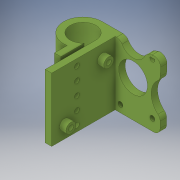
# Autodesk Inventor part: motor mount 2
Saved by Autodesk Inventor 2018 (Build 220112000, 112)
## iProperties
Created: 2017-11-21
Part Number: motor mount 2
Material: ABS Plastic
Document SubType Name: Modeling
Designer: prakhar
Density: 1.06 g/cm^3
Appearance: Olive Green
Author: prakhar
Autodesk Inventor part; units mm, degrees
ref_plane "YZ Plane" through (0, 0, 0) normal (1, 0, 0) x (0, 1, 0)
ref_plane "XZ Plane" through (0, 0, 0) normal (0, 1, 0) x (-1, 0, 0)
ref_plane "XY Plane" through (0, 0, 0) normal (0, 0, 1) x (1, 0, 0)
sketch "Sketch1" plane through (0, 0, 0) normal (1, 0, 0) x (0, 1, 0)
  line L0 (19.8793, 20.7795) -> (-17.4785, 20.7795)
  line L1 (-17.4785, 20.7795) -> (-17.4785, -16.5784)
  line L2 (-17.4785, -16.5784) -> (19.8793, -16.5784)
  line L3 (19.8793, -16.5784) -> (19.8793, 20.7795)
  circle A0 centre (19.8793, 20.7795) radius 4.8895
  circle A1 centre (19.8793, -16.5784) radius 4.8895
  circle A2 centre (-17.4785, -16.5784) radius 4.8895
  circle A3 centre (-17.4785, 20.7795) radius 4.8895
  line L4 (32.5793, 33.4795) -> (-30.1785, 33.4795)
  line L5 (-30.1785, 33.4795) -> (-30.1785, -29.2784)
  line L6 (-30.1785, -29.2784) -> (32.5793, -29.2784)
  line L7 (32.5793, -29.2784) -> (32.5793, 33.4795)
  circle A4 centre (19.8793, 20.7795) radius 2.4575
  circle A5 centre (19.8793, -16.5784) radius 2.4575
  circle A6 centre (-17.4785, -16.5784) radius 2.4575
  circle A7 centre (-17.4785, 20.7795) radius 2.4575
  point P0 (0, 0)
  dimension "d0" = 9.779
  dimension "d4" = 52.832
  dimension "d5" = 12.7
  dimension "d6" = 12.7
  dimension "d7" = 12.7
  dimension "d8" = 12.7
  dimension "d13" = 4.9149
  constraints: 16 end point, 8 centre point, 8 coincident, 6 equal radius, 4 parallel, 3 perpendicular, 2 horizontal
  measures "d0" diameter of A2
  measures "d4" distance of L2.end L0.end
  measures "d5" distance from line of L0.end L5
  measures "d6" distance between parallel lines of L4 L0
  measures "d7" distance between parallel lines of L7 L3
  measures "d8" distance between parallel lines of L6 L2
  measures "d13" diameter of A4
extrude "Extrusion1" add sketch "Sketch1" along normal blind 6.35 contours A3 L1 A7 L0 | L0 A7 L1 A3 | L0 A0 L3 A1 L2 A2 L1 A3 | A7 L1 L0 | L0 L1 A7 | A0 L3 A4 L0 | L0 A4 L3 A0 | A4 L3 L0 | L0 L3 A4 | A2 L2 A6 L1 | L1 A6 L2 A2 | A1 L2 A5 L3 | L3 A5 L2 A1 | A6 L2 L1 | L1 L2 A6 | A5 L2 L3 | L3 L2 A5 | L7 L6 L5 L4
extrude "Extrusion2" add sketch "Sketch1" along normal blind 12.7 contours A3 L1 A7 L0 | L0 A7 L1 A3 | A7 L1 L0 | L0 L1 A7 | A1 L2 A5 L3 | L3 A5 L2 A1 | A5 L2 L3 | L3 L2 A5
extrude "Extrusion3" cut sketch "Sketch1" along normal blind 12.7 contours A7 L1 L0 | L0 L1 A7 | A5 L2 L3 | L3 L2 A5
sketch "Sketch2" plane through (0, -30.1785, -29.2784) normal (0, 0, -1) x (-1, 0, 0)
  line L0 (0, 0) -> (-6.35, 0) projected
  line L1 (0, 0) -> (-50.8, 0)
  line L2 (-50.8, 0) -> (-50.8, 62.7579)
  line L3 (-50.8, 62.7579) -> (0, 62.7579)
  line L4 (0, 62.7579) -> (0, 0)
  line L5 (0, 62.7579) -> (-6.35, 62.7579) projected
  arc A0 (-36.4267, 62.7579) -> (-11.8333, 62.7579) centre (-24.13, 65.9329) ccw
  point P0 (0, 30.1785)
  dimension "d16" = 50.8
  dimension "d30" = 12.7
  dimension "d31" = 24.13
  dimension "d32" = 3.175
  constraints: 8 end point, 2 parallel, 2 point on circle, 2 point on line, 1 centre point, 1 collinear, 1 horizontal, 1 perpendicular
  measures "d16" distance of L2.end L3.end
  measures "d30" radius of A0
  measures "d31" distance from line of A0.centre L4
  measures "d32" distance from line of A0.centre L3
extrude "Extrusion4" add sketch "Sketch2" along normal blind 6.35 contours L0 L1 L2 L3 A0 L4
sketch "Sketch4" plane through (0, 32.5793, 33.4795) normal (0, 1, 0) x (1, 0, 0)
  line L0 (0, 0) -> (0, 69.1079) projected
  line L1 (0, 0) -> (6.35, 0) projected
  line L2 (6.35, 62.7579) -> (6.35, 0) projected
  line L3 (36.4267, 62.7579) -> (50.8, 62.7579) projected
  line L4 (50.8, 62.7579) -> (50.8, 69.1079) projected
  line L5 (36.4267, 69.1079) -> (50.8, 69.1079) projected
  line L6 (0, 69.1079) -> (6.35, 69.1079)
  line L7 (6.35, 69.1079) -> (6.35, 119.9079)
  line L8 (6.35, 119.9079) -> (0, 119.9079)
  line L9 (0, 119.9079) -> (0, 69.1079)
  line L10 (6.35, 119.9079) -> (50.8, 119.9079)
  line L11 (50.8, 119.9079) -> (50.8, 113.5579)
  line L12 (50.8, 113.5579) -> (6.35, 113.5579)
  line L13 (6.35, 113.5579) -> (6.35, 119.9079)
  line L14 (6.35, 62.7579) -> (11.8333, 62.7579) projected
  line L15 (11.8333, 62.7579) -> (11.8333, 69.1079) projected
  line L16 (0, 69.1079) -> (11.8333, 69.1079) projected
  line L17 (36.4267, 62.7579) -> (36.4267, 69.1079) projected
  point P0 (0, 33.4795)
  dimension "d25" = 6.35
  dimension "d26" = 50.8
  dimension "d27" = 6.35
  constraints: 16 end point, 4 parallel, 2 horizontal, 2 perpendicular, 1 collinear
  measures "d25" distance of L10.end L11.end
  measures "d26" distance of L6.end L7.end
  measures "d27" distance between parallel lines of L9 L7
sketch "Sketch3" plane through (0, -30.1785, -29.2784) normal (0, 0, 1) x (1, 0, 0)
  circle A0 centre (24.1046, 36.4435) radius 9.7536
  line L0 (6.35, 62.7579) -> (6.35, 0) projected
  line L1 (6.35, 62.7579) -> (50.8, 62.7579) projected
  circle A1 centre (24.1046, 36.4435) radius 14.2494
  point P0 (0, 30.1785)
  dimension "d19" = 19.5072
  dimension "d20" = 17.7546
  dimension "d21" = 26.3144
  dimension "d22" = 28.4988
  constraints: 2 centre point, 1 coincident
  measures "d19" diameter of A0
  measures "d20" distance from line of A0.centre L0
  measures "d21" distance from line of A0.centre L1
  measures "d22" diameter of A1
extrude "Extrusion5" cut sketch "Sketch3" against normal blind 63.5 contours A0 | A1
sketch "Sketch5" plane through (0, -30.1785, -29.2784) normal (0, 0, 1) x (1, 0, 0)
  circle A0 centre (24.1046, 36.4435) radius 14.2494 projected
  circle A1 centre (43.1546, 61.8435) radius 2.4574
  circle A2 centre (43.1546, 11.0435) radius 2.4574
  circle A3 centre (11.6326, 7.2457) radius 2.4574
  point P0 (0, 30.1785)
  dimension "d33" = 4.9149
  dimension "d46" = 31.75
  dimension "d47" = 31.75
  dimension "d48" = 31.75
  dimension "d49" = 31.75
  dimension "d50" = 50.8
  dimension "d51" = 25.4
  constraints: 3 centre point, 2 equal radius
  measures "d33" diameter of A2
  measures "d46" distance of A0.centre A1.centre
  measures "d47" distance of A0.centre A2.centre
  measures "d48" distance of A0.centre A3.centre
  measures "d49" distance of A2.centre A3.centre
  measures "d50" distance of A1.centre A2.centre
  measures "d51" vertical distance of A0.centre A2.centre
extrude "Extrusion7" cut sketch "Sketch5" against normal blind 25.4 contours A1 | A2 | A3
sketch "Sketch6" plane through (0, -30.1785, -29.2784) normal (0, 0, 1) x (1, 0, 0)
  line L0 (50.8, 62.7579) -> (50.8, 0) projected
  arc A0 (50.8, 47.8645) -> (50.8, 15.6355) centre (60.96, 31.75) ccw
  line L1 (50.8, 47.8645) -> (50.8, 15.6355)
  line L2 (50.8, 0) -> (6.35, 0) projected
  point P0 (0, 30.1785)
  dimension "d40" = 19.05
  dimension "d41" = 31.75
  dimension "d42" = 10.16
  constraints: 2 end point, 2 point on circle, 1 centre point, 1 collinear, 1 point on line
  measures "d40" radius of A0
  measures "d41" distance from line of L2 A0.centre
  measures "d42" distance from line of L0 A0.centre
extrude "Extrusion8" cut sketch "Sketch6" against normal blind 25.4
sketch "Sketch7" plane through (0, -30.1785, -29.2784) normal (0, 0, 1) x (1, 0, 0)
  line L0 (50.8, 62.7579) -> (50.8, 47.8645) projected
  line L1 (36.4267, 62.7579) -> (50.8, 62.7579) projected
  line L2 (50.8, 47.8645) -> (51.4653, 68.2507)
  line L3 (51.4653, 68.2507) -> (36.4267, 62.7579)
  point P0 (0, 30.1785)
  constraints: 4 end point
extrude "Extrusion9" add sketch "Sketch7" against normal up to surface (6.35 mm away)
fillet "Fillet2" radius 6.35 6 edges at (36.4267, 32.5793, -32.4534) (11.8333, 32.5793, -32.4534) (51.4653, 38.0722, -32.4534) (50.8, 17.686, -32.4534) (50.8, -14.543, -32.4534) (50.8, -30.1785, -32.4534)
sketch "Sketch8" plane through (0, -30.1785, 33.4795) normal (0, -1, 0) x (1, 0, 0)
  arc A0 (-3.175, -41.6576) -> (0, -50.0579) centre (-12.7, -50.0579) ccw
  line L0 (44.45, -69.1079) -> (0, -69.1079) projected
  line L1 (0, 0) -> (0, -69.1079) projected
  line L2 (0, -69.1079) -> (-12.7, -69.1079)
  line L3 (-3.175, -41.6576) -> (-3.175, -18.5743)
  line L4 (-3.175, -18.5743) -> (-9.525, -18.5743)
  line L5 (-9.525, -18.5743) -> (-9.525, -31.2743)
  arc A1 (-9.525, -31.2743) -> (-12.7, -69.1079) centre (-12.7, -50.0579) ccw
  point P0 (0, -33.4795)
  dimension "d57" = 25.4
  dimension "d59" = 19.05
  dimension "d60" = 6.35
  dimension "d61" = 3.175
  dimension "d62" = 12.7
  constraints: 8 end point, 4 point on circle, 2 centre point, 2 tangent, 1 coincident, 1 horizontal, 1 parallel, 1 perpendicular, 1 point on line
  measures "d57" diameter of A0
  measures "d59" radius of A1
  measures "d60" distance of L3.end L4.end
  measures "d61" distance between parallel lines of L1 L3
  measures "d62" distance of L4.end L5.end
extrude "Extrusion10" add sketch "Sketch8" against normal up to surface (62.7579 mm away)
sketch "Sketch9" plane through (-9.525, -30.1785, 2.2051) normal (-1, 0, 0) x (0, 0, 1)
  circle A0 centre (6.35, 56.4079) radius 2.54
  line L0 (12.7, 0) -> (12.7, 62.7579) projected
  line L1 (12.7, 62.7579) -> (0, 62.7579) projected
  circle A1 centre (6.35, 43.7079) radius 2.54
  circle A2 centre (6.35, 31.0079) radius 2.54
  circle A3 centre (6.35, 18.3079) radius 2.54
  circle A4 centre (6.35, 5.6079) radius 2.54
  point P0 (-2.2051, 30.1785)
  dimension "d65" = 6.35
  dimension "d66" = 6.35
  dimension "d67" = 5.08
  dimension "d70" = 12.7
  constraints: 5 centre point, 1 vertical, 8 other
  measures "d65" distance from line of L0 A0.centre
  measures "d66" distance from line of A0.centre L1
  measures "d67" diameter of A0
  measures "d70" distance of A0.centre A1.centre
extrude "Extrusion11" cut sketch "Sketch9" against normal up to surface (6.35 mm away)
sketch "Sketch10" plane through (0, 0, 0) normal (-1, 0, 0) x (0, 0, 1)
  line L0 (14.9051, -30.1785) -> (14.9051, 32.5793) projected
  line L1 (14.9051, 32.5793) -> (2.2051, 32.5793) projected
  circle A0 centre (8.5551, 26.2293) radius 2.4574
  circle A1 centre (8.5551, 13.5293) radius 2.4574
  circle A2 centre (8.5551, 0.8293) radius 2.4574
  circle A3 centre (8.5551, -11.8707) radius 2.4574
  circle A4 centre (8.5551, -24.5707) radius 2.4574
  point P0 (0, 0)
  dimension "d77" = 4.9149
  dimension "d78" = 6.35
  dimension "d79" = 6.35
  dimension "d82" = 12.7
  constraints: 5 centre point, 1 vertical, 8 other
  measures "d77" diameter of A0
  measures "d78" distance from line of L0 A0.centre
  measures "d79" distance from line of A0.centre L1
  measures "d82" distance of A0.centre A1.centre
extrude "Extrusion12" cut sketch "Sketch10" against normal blind 25.4
equation "\"d27\" = d25"
equation "\"d1\" = d0"
body "Solid1"
